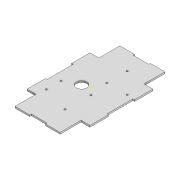
# Autodesk Inventor part: 본체 밑판 레이저 수정
Saved by Autodesk Inventor 2020 (Build 240168000, 168)
## iProperties
Created: 2022-08-25
Part Number: 본체 밑판 레이저 수정
Material: 일반
Document SubType Name: Modeling
Designer: 박연호
Density: 1 g/cm^3
Appearance: 기본값
Author: 박연호
Autodesk Inventor part; units mm, degrees
ref_plane "YZ Plane" through (0, 0, 0) normal (1, 0, 0) x (0, 1, 0)
ref_plane "XZ Plane" through (0, 0, 0) normal (0, 1, 0) x (-1, 0, 0)
ref_plane "XY Plane" through (0, 0, 0) normal (0, 0, 1) x (1, 0, 0)
sketch "스케치1" plane through (0, 0, 0) normal (0, 1, 0) x (-1, 0, 0)
  line L0 (60, -100) -> (-60, -100)
  line L1 (-60, -100) -> (-60, 100)
  line L2 (-60, 100) -> (60, 100)
  line L3 (60, 100) -> (60, -100)
  line L4 (60, -100) -> (-60, 100) construction
  line L5 (-60, -100) -> (60, 100) construction
  point P0 (0, 0)
  dimension "d0" = 200
  dimension "d1" = 120
  constraints: 12 end point, 2 midpoint, 2 parallel, 1 horizontal, 1 perpendicular
  measures "d0" distance of L2.end L0.start
  measures "d1" distance of L1.end L2.end
extrude "돌출1" add sketch "스케치1" along normal blind 3
sketch "스케치3" plane through (0, 3, 0) normal (0, 1, 0) x (1, 0, 0)
  line L0 (-43.6, -60) -> (25, -60)
  line L1 (25, -60) -> (25, -6.6)
  line L2 (25, -6.6) -> (-43.6, -6.6)
  line L3 (-43.6, -6.6) -> (-43.6, -60)
  circle A0 centre (9.7, -57.45) radius 1.6
  circle A1 centre (11.03, -9.15) radius 1.6
  circle A2 centre (-41.05, -42.16) radius 1.6
  circle A3 centre (-41.05, -14.23) radius 1.6
  line L4 (60, -100) -> (60, 100) projected
  line L5 (-60, -100) -> (60, -100) projected
  point P0 (0, 0)
  point P1 (0, 0)
  dimension "d22" = 68.6
  dimension "d23" = 53.4
  dimension "d26" = 3.2
  dimension "d27" = 15.3
  dimension "d28" = 2.55
  dimension "d29" = 3.2
  dimension "d30" = 13.97
  dimension "d31" = 2.55
  dimension "d32" = 3.2
  dimension "d33" = 35.56
  dimension "d34" = 3.2
  dimension "d35" = 2.55
  dimension "d36" = 2.55
  dimension "d37" = 7.63
  dimension "d38" = 35
  dimension "d40" = 40
  constraints: 8 end point, 4 centre point, 2 parallel, 1 horizontal, 1 perpendicular
  measures "d22" distance of L1.end L2.end
  measures "d23" distance of L2.end L0.start
  measures "d26" diameter of A0
  measures "d27" distance from line of L1 A0.centre
  measures "d28" distance from line of A0.centre L0
  measures "d29" diameter of A1
  measures "d30" distance from line of L1 A1.centre
  measures "d31" distance from line of L2 A1.centre
  measures "d32" diameter of A2
  measures "d33" distance from line of L2 A2.centre
  measures "d34" diameter of A3
  measures "d35" distance from line of L3 A3.centre
  measures "d36" distance from line of L3 A2.centre
  measures "d37" distance from line of L2 A3.centre
  measures "d38" distance between parallel lines of L4 L1
  measures "d40" distance between parallel lines of L5 L0
extrude "돌출2" cut sketch "스케치3" against normal through all contours A0 | A1 | A2 | A3
sketch "스케치4" plane through (0, 3, 0) normal (0, 1, 0) x (1, 0, 0)
  line L0 (6, 26) -> (45, 26)
  line L1 (45, 26) -> (45, 65)
  line L2 (45, 65) -> (6, 65)
  line L3 (6, 65) -> (6, 26)
  circle A0 centre (6, 26) radius 1.6
  circle A1 centre (6, 65) radius 1.6
  circle A2 centre (45, 65) radius 1.6
  circle A3 centre (45, 26) radius 1.6
  line L4 (-47.9371, 14.7215) -> (-7.9371, 14.7215)
  line L5 (-7.9371, 14.7215) -> (-7.9371, 64.7215)
  line L6 (-7.9371, 64.7215) -> (-47.9371, 64.7215)
  line L7 (-47.9371, 64.7215) -> (-47.9371, 14.7215)
  line L8 (60, -100) -> (60, 100) projected
  line L9 (60, 100) -> (-60, 100) projected
  circle A4 centre (-15, -1) radius 10
  line L10 (-60, 100) -> (-60, -100) projected
  point P0 (0, 0)
  point P1 (0, 0)
  dimension "d43" = 39
  dimension "d44" = 39
  dimension "d47" = 3.2
  dimension "d48" = 3.2
  dimension "d49" = 3.2
  dimension "d50" = 3.2
  dimension "d51" = 40
  dimension "d52" = 50
  dimension "d53" = 15
  dimension "d54" = 35
  dimension "d56" = 20
  dimension "d69" = 45
  dimension "d70" = 101
  constraints: 16 end point, 5 centre point, 4 coincident, 4 parallel, 2 horizontal, 2 perpendicular
  measures "d43" distance of L2.end L0.start
  measures "d44" distance of L1.end L2.end
  measures "d47" diameter of A0
  measures "d48" diameter of A1
  measures "d49" diameter of A2
  measures "d50" diameter of A3
  measures "d51" distance of L5.end L6.end
  measures "d52" distance of L6.end L4.start
  measures "d53" distance between parallel lines of L8 L1
  measures "d54" distance between parallel lines of L9 L2
  measures "d56" diameter of A4
  measures "d69" distance from line of A4.centre L10
  measures "d70" distance from line of L9 A4.centre
extrude "돌출3" cut sketch "스케치4" against normal through all contours L3 A0 L0 | L0 A0 L3 | A3 L1 L0 | L0 L1 A3 | A1 L2 L3 | L3 L2 A1 | A2 L2 L1 | L1 L2 A2 | A4
sketch "스케치5" plane through (0, 3, 0) normal (0, 1, 0) x (1, 0, 0)
  line L0 (57, -25) -> (61.988, -25)
  line L1 (61.988, -25) -> (61.988, 25)
  line L2 (61.988, 25) -> (57, 25)
  line L3 (57, 25) -> (57, -25)
  line L4 (60, -100) -> (60, 100) projected
  line L5 (60, 100) -> (-60, 100) projected
  line L6 (0, -100) -> (0, 100)
  line L7 (60, 100) -> (-60, 100) projected
  line L8 (-57, -25) -> (-61.988, -25)
  line L9 (-61.988, -25) -> (-61.988, 25)
  line L10 (-61.988, 25) -> (-57, 25)
  line L11 (-57, 25) -> (-57, -25)
  point P0 (0, 0)
  dimension "d59" = 50
  dimension "d60" = 3
  dimension "d61" = 75
  constraints: 18 end point, 4 symmetric about line, 2 parallel, 1 horizontal, 1 midpoint, 1 perpendicular
  measures "d59" distance of L0.end L1.end
  measures "d60" distance between parallel lines of L4 L3
  measures "d61" distance between parallel lines of L5 L2
extrude "돌출4" cut sketch "스케치5" against normal through all
sketch "스케치6" plane through (0, 3, 0) normal (0, 1, 0) x (1, 0, 0)
  line L0 (-15, -110.8891) -> (15, -110.8891)
  line L1 (15, -110.8891) -> (15, -97)
  line L2 (15, -97) -> (-15, -97)
  line L3 (-15, -97) -> (-15, -110.8891)
  line L4 (-60, -100) -> (60, -100) projected
  line L5 (-60, -25) -> (-60, -100) projected
  line L6 (-57, -25) -> (-57, 25) projected
  line L7 (-57, 0) -> (56.7319, 0)
  line L8 (-15, 110.8891) -> (15, 110.8891)
  line L9 (15, 110.8891) -> (15, 97)
  line L10 (15, 97) -> (-15, 97)
  line L11 (-15, 97) -> (-15, 110.8891)
  point P0 (0, 0)
  dimension "d64" = 30
  dimension "d65" = 3
  dimension "d66" = 45
  constraints: 18 end point, 4 symmetric about line, 2 horizontal, 2 parallel, 1 midpoint, 1 perpendicular
  measures "d64" distance of L0.start L0.end
  measures "d65" distance between parallel lines of L2 L4
  measures "d66" distance between parallel lines of L5 L3
extrude "돌출5" cut sketch "스케치6" against normal through all
sketch "스케치7" plane through (0, 3, 0) normal (0, 1, 0) x (1, 0, 0)
  point P0 (0, 0)
sketch "스케치8" plane through (0, 0, 0) normal (0, -1, 0) x (1, 0, 0)
  line L0 (60, 100) -> (60, 25) projected
  line L1 (60, 100) -> (43, 100)
  line L2 (43, 100) -> (43, 60)
  line L3 (43, 60) -> (60, 60)
  line L4 (60, 60) -> (60, 100)
  line L5 (57, -25) -> (57, 25) projected
  line L6 (57, 0) -> (-57, 0)
  line L7 (-57, 25) -> (-57, -25) projected
  line L8 (15, 97) -> (-15, 97) projected
  line L9 (0, 97) -> (0, -97)
  line L10 (15, -97) -> (-15, -97) projected
  line L11 (-60, 100) -> (-43, 100)
  line L12 (-43, 100) -> (-43, 60)
  line L13 (-43, 60) -> (-60, 60)
  line L14 (-60, 25) -> (-60, 100) projected
  line L15 (60, -25) -> (60, -100) projected
  line L16 (-60, -100) -> (-60, -25) projected
  line L17 (-15, -100) -> (-60, -100) projected
  line L18 (60, -100) -> (15, -100) projected
  line L19 (60, -100) -> (43, -100)
  line L20 (43, -100) -> (43, -60)
  line L21 (43, -60) -> (60, -60)
  line L22 (60, -60) -> (60, -100)
  line L23 (-60, -100) -> (-43, -100)
  line L24 (-43, -100) -> (-43, -60)
  line L25 (-43, -60) -> (-60, -60)
  point P0 (0, 0)
  dimension "d71" = 17
  dimension "d72" = 40
  constraints: 32 end point, 10 symmetric about line, 4 midpoint, 2 parallel, 1 horizontal, 1 perpendicular
  measures "d71" distance of L0.start L1.end
  measures "d72" distance of L1.end L2.end
extrude "돌출6" cut sketch "스케치8" against normal through all
